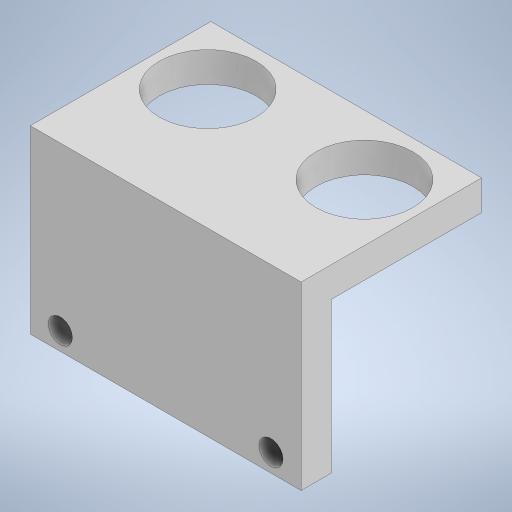
# Autodesk Inventor part: distance sensor
Saved by Autodesk Inventor 2024 (Build 280153000, 153)
## iProperties
Created: 2024-10-01
Part Number: distance sensor
Material: Všeobecné
Document SubType Name: Modeling
Designer: elias
Density: 1 g/cm^3
Appearance: Výchozí
Author: elias
Autodesk Inventor part; units mm, degrees
ref_plane "YZ Plane" through (0, 0, 0) normal (1, 0, 0) x (0, 1, 0)
ref_plane "XZ Plane" through (0, 0, 0) normal (0, 1, 0) x (-1, 0, 0)
ref_plane "XY Plane" through (0, 0, 0) normal (0, 0, 1) x (1, 0, 0)
sketch "Náčrt1" plane through (0, 0, 0) normal (0, 0, 1) x (1, 0, 0)
  circle A0 centre (13.025, 0) radius 8.05
  circle A1 centre (-13.025, 0) radius 8.05
  line L0 (22.5, 0) -> (22.5, 10)
  line L1 (22.5, 10) -> (-22.5, 10)
  line L2 (-22.5, 10) -> (-22.5, -20)
  line L3 (-22.5, -20) -> (22.5, -20)
  line L4 (22.5, -20) -> (22.5, 0)
  point P0 (0, 0)
  point P1 (0, 0)
  dimension "d2" = 16.1
  dimension "d5" = 10
  dimension "d6" = 30
  dimension "d18" = 16.1
  constraints: 10 end point, 2 centre point, 2 perpendicular, 2 vertical, 1 horizontal
  measures "d2" diameter of A0
  measures "d5" distance of L0.start L0.end
  measures "d6" distance of L1.end L2.end
  measures "d18" diameter of A1
extrude "Vysunutí1" add sketch "Náčrt1" along normal blind 5
sketch "Náčrt2" plane through (0, 0, 0) normal (0, 0, -1) x (-1, 0, 0)
  line L0 (-22.5, -20) -> (-22.5, 10) projected
  line L1 (-22.5, -20) -> (22.5, -20)
  line L2 (22.5, -20) -> (22.5, -15)
  line L3 (22.5, -15) -> (-22.5, -15)
  line L4 (-22.5, -15) -> (-22.5, -20)
  point P0 (0, 0)
  dimension "d9" = 45
  dimension "d10" = 5
  constraints: 8 end point, 2 parallel, 1 horizontal, 1 perpendicular
  measures "d9" distance of L3.end L2.end
  measures "d10" distance of L1.end L2.end
extrude "Vysunutí2" add sketch "Náčrt2" along normal blind 25
sketch "Náčrt3" plane through (-22.5, -15, 0) normal (0, 1, 0) x (1, 0, 0)
  circle A0 centre (40, 22) radius 2
  line L0 (45, 0) -> (45, 25) projected
  line L1 (0, 25) -> (45, 25) projected
  line L2 (22.5, 25) -> (22.5, 18.3064)
  circle A1 centre (5, 22) radius 2
  point P0 (22.5, 0)
  dimension "d13" = 4
  dimension "d14" = 5
  dimension "d15" = 3
  constraints: 2 centre point, 2 end point, 1 midpoint, 1 symmetric about line, 1 vertical, 1 other
  measures "d13" diameter of A0
  measures "d14" distance from line of L0 A0.centre
  measures "d15" distance from line of A0.centre L1
extrude "Vysunutí3" cut sketch "Náčrt3" against normal blind 25
